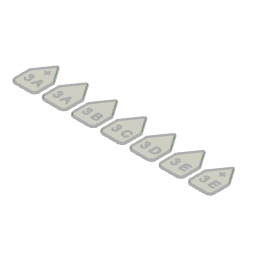
_Pointed Markers 3s.d0f4be62-6763-4f03-b29f-435d984270f3 (Autodesk Fusion 360 design; units mm, degrees)
Autodesk Fusion 360 part; units mm, degrees
sketch "Sketch1" plane through (0, 0, 0) normal (0, 0, 1) x (1, 0, 0)
  line L0 (0, 50.8) -> (0, 0)
  arc A0 (-31.7281, 6.3281) -> (-25.4, 0) centre (-25.4, 6.3281) ccw
  line L1 (-25.4, 0) -> (-15.875, 0)
  line L2 (-31.7281, 25.3781) -> (-31.7281, 6.3281)
  line L3 (-31.7281, 25.3781) -> (-15.7092, 48.2556)
  line L4 (-6.0183, 0) -> (-15.5433, 0)
  line L5 (0.3098, 25.3781) -> (-15.7092, 48.2556)
  arc A1 (-6.0183, 0) -> (0.3098, 6.3281) centre (-6.0183, 6.3281) ccw
  line L6 (0.3098, 25.3781) -> (0.3098, 6.3281)
  line L7 (-15.875, 0) -> (-15.5433, 0)
  dimension "d4" = 50.8
  dimension "d12" = 19.05
  constraint vertical L0
  constraint coincident L0.end origin
  constraint tangent A0 L1
  constraint vertical L2
  constraint parallel L4 L7
  measures "d4" distance of L0.end L0.start
  measures "d12" distance of A0.start L2.start
extrude "Extrude1" add sketch "Sketch1" along normal blind 1 contours L0 A0 L1 L2 L3 L4 L5 A1 L7 makes body 1
fillet "Fillet1" radius 2 3 edges at (0, 25.8206, 0.5) (-31.7281, 25.3781, 0.5) (-15.7092, 48.2556, 0.5) on bodies 1
sketch "Sketch2" plane through (0, 0, 1) normal (0, 0, 1) x (-1, 0, 0)
  arc A0 (14.0709, -45.9158) -> (17.3475, -45.9158) centre (15.7092, -44.7687) ccw
  line L0 (17.3475, -45.9158) -> (31.3664, -25.8947)
  arc A1 (31.3664, -25.8947) -> (31.7281, -24.7475) centre (29.7281, -24.7475) ccw
  line L1 (31.7281, -24.7475) -> (31.7281, -6.3281)
  arc A2 (31.7281, -6.3281) -> (25.4, 0) centre (25.4, -6.3281) ccw
  line L2 (25.4, 0) -> (6.0183, 0)
  arc A3 (6.0183, 0) -> (0, -4.3724) centre (6.0183, -6.3281) ccw
  line L3 (0, -4.3724) -> (0, -25.19)
  arc A4 (0, -25.19) -> (0.3617, -26.3371) centre (2, -25.19) ccw
  line L4 (0.3617, -26.3371) -> (14.0709, -45.9158)
  line L5 (16.1187, -45.0555) -> (30.1377, -25.0343)
  arc A5 (30.1377, -25.0343) -> (30.2281, -24.7475) centre (29.7281, -24.7475) ccw
  line L6 (30.2281, -24.7475) -> (30.2281, -6.3281)
  arc A6 (30.2281, -6.3281) -> (25.4, -1.5) centre (25.4, -6.3281) ccw
  line L7 (25.4, -1.5) -> (6.0183, -1.5)
  arc A7 (6.0183, -1.5) -> (1.5, -4.6265) centre (6.0183, -6.3281) ccw
  line L8 (1.5, -4.6265) -> (1.5, -25.19)
  arc A8 (1.5, -25.19) -> (1.5904, -25.4768) centre (2, -25.19) ccw
  line L9 (1.5904, -25.4768) -> (15.2996, -45.0555)
  arc A9 (15.2996, -45.0555) -> (16.1187, -45.0555) centre (15.7092, -44.7687) ccw
  line L10 (25.6864, -13.7884) -> (3.6261, -13.7884) construction
  line L11 (3.6261, -13.7884) -> (3.6261, -25.3842) construction
  line L12 (3.6261, -25.3842) -> (25.6864, -25.3842) construction
  line L13 (25.6864, -25.3842) -> (25.6864, -13.7884) construction
  dimension "d18" = -1.5
  dimension "d19" = 10.0076
copy_body "Body->Comp1" bodies 1 removing the originals makes body 2 in component "Arrow Base"
pattern_linear "R-Pattern1" count 1 spacing 0 along (0, 1, 0) count 7 spacing 38.1 along (1, 0, 0) of bodies 2 makes body 3 at (19.0573, 16.6458, 0) makes body 4 at (57.1573, 16.6458, 0) makes body 5 at (95.2573, 16.6458, 0) makes body 6 at (133.3573, 16.6458, 0) makes body 7 at (171.4573, 16.6458, 0) makes body 8 at (209.5573, 16.6458, 0) in component "Arrow Base"
sketch "Sketch3" plane through (0, 0, 1) normal (0, 0, 1) x (-1, 0, 0)
  arc A0 (14.0709, -45.9158) -> (17.3475, -45.9158) centre (15.7092, -44.7687) ccw
  line L0 (17.3475, -45.9158) -> (31.3664, -25.8947)
  arc A1 (31.3664, -25.8947) -> (31.7281, -24.7475) centre (29.7281, -24.7475) ccw
  line L1 (31.7281, -24.7475) -> (31.7281, -6.3281)
  arc A2 (31.7281, -6.3281) -> (25.4, 0) centre (25.4, -6.3281) ccw
  line L2 (25.4, 0) -> (6.0183, 0)
  arc A3 (6.0183, 0) -> (0, -4.3724) centre (6.0183, -6.3281) ccw
  line L3 (0, -4.3724) -> (0, -25.19)
  arc A4 (0, -25.19) -> (0.3617, -26.3371) centre (2, -25.19) ccw
  line L4 (0.3617, -26.3371) -> (14.0709, -45.9158)
  arc A5 (-24.0291, -45.9158) -> (-20.7525, -45.9158) centre (-22.3908, -44.7687) ccw
  line L5 (-20.7525, -45.9158) -> (-6.7336, -25.8947)
  arc A6 (-6.7336, -25.8947) -> (-6.3719, -24.7475) centre (-8.3719, -24.7475) ccw
  line L6 (-6.3719, -24.7475) -> (-6.3719, -6.3281)
  arc A7 (-6.3719, -6.3281) -> (-12.7, 0) centre (-12.7, -6.3281) ccw
  line L7 (-12.7, 0) -> (-32.0817, 0)
  arc A8 (-32.0817, 0) -> (-38.1, -4.3724) centre (-32.0817, -6.3281) ccw
  line L8 (-38.1, -4.3724) -> (-38.1, -25.19)
  arc A9 (-38.1, -25.19) -> (-37.7383, -26.3371) centre (-36.1, -25.19) ccw
  line L9 (-37.7383, -26.3371) -> (-24.0291, -45.9158)
  arc A10 (-62.1291, -45.9158) -> (-58.8525, -45.9158) centre (-60.4908, -44.7687) ccw
  line L10 (-58.8525, -45.9158) -> (-44.8336, -25.8947)
  arc A11 (-44.8336, -25.8947) -> (-44.4719, -24.7475) centre (-46.4719, -24.7475) ccw
  line L11 (-44.4719, -24.7475) -> (-44.4719, -6.3281)
  arc A12 (-44.4719, -6.3281) -> (-50.8, 0) centre (-50.8, -6.3281) ccw
  line L12 (-50.8, 0) -> (-70.1817, 0)
  arc A13 (-70.1817, 0) -> (-76.2, -4.3724) centre (-70.1817, -6.3281) ccw
  line L13 (-76.2, -4.3724) -> (-76.2, -25.19)
  arc A14 (-76.2, -25.19) -> (-75.8383, -26.3371) centre (-74.2, -25.19) ccw
  line L14 (-75.8383, -26.3371) -> (-62.1291, -45.9158)
  arc A15 (-100.2291, -45.9158) -> (-96.9525, -45.9158) centre (-98.5908, -44.7687) ccw
  line L15 (-96.9525, -45.9158) -> (-82.9336, -25.8947)
  arc A16 (-82.9336, -25.8947) -> (-82.5719, -24.7475) centre (-84.5719, -24.7475) ccw
  line L16 (-82.5719, -24.7475) -> (-82.5719, -6.3281)
  arc A17 (-82.5719, -6.3281) -> (-88.9, 0) centre (-88.9, -6.3281) ccw
  line L17 (-88.9, 0) -> (-108.2817, 0)
  arc A18 (-108.2817, 0) -> (-114.3, -4.3724) centre (-108.2817, -6.3281) ccw
  line L18 (-114.3, -4.3724) -> (-114.3, -25.19)
  arc A19 (-114.3, -25.19) -> (-113.9383, -26.3371) centre (-112.3, -25.19) ccw
  line L19 (-113.9383, -26.3371) -> (-100.2291, -45.9158)
  arc A20 (-138.3291, -45.9158) -> (-135.0525, -45.9158) centre (-136.6908, -44.7687) ccw
  line L20 (-135.0525, -45.9158) -> (-121.0336, -25.8947)
  arc A21 (-121.0336, -25.8947) -> (-120.6719, -24.7475) centre (-122.6719, -24.7475) ccw
  line L21 (-120.6719, -24.7475) -> (-120.6719, -6.3281)
  arc A22 (-120.6719, -6.3281) -> (-127, 0) centre (-127, -6.3281) ccw
  line L22 (-127, 0) -> (-146.3817, 0)
  arc A23 (-146.3817, 0) -> (-152.4, -4.3724) centre (-146.3817, -6.3281) ccw
  line L23 (-152.4, -4.3724) -> (-152.4, -25.19)
  arc A24 (-152.4, -25.19) -> (-152.0383, -26.3371) centre (-150.4, -25.19) ccw
  line L24 (-152.0383, -26.3371) -> (-138.3291, -45.9158)
  arc A25 (-176.4291, -45.9158) -> (-173.1525, -45.9158) centre (-174.7908, -44.7687) ccw
  line L25 (-173.1525, -45.9158) -> (-159.1336, -25.8947)
  arc A26 (-159.1336, -25.8947) -> (-158.7719, -24.7475) centre (-160.7719, -24.7475) ccw
  line L26 (-158.7719, -24.7475) -> (-158.7719, -6.3281)
  arc A27 (-158.7719, -6.3281) -> (-165.1, 0) centre (-165.1, -6.3281) ccw
  line L27 (-165.1, 0) -> (-184.4817, 0)
  arc A28 (-184.4817, 0) -> (-190.5, -4.3724) centre (-184.4817, -6.3281) ccw
  line L28 (-190.5, -4.3724) -> (-190.5, -25.19)
  arc A29 (-190.5, -25.19) -> (-190.1383, -26.3371) centre (-188.5, -25.19) ccw
  line L29 (-190.1383, -26.3371) -> (-176.4291, -45.9158)
  arc A30 (-214.5291, -45.9158) -> (-211.2525, -45.9158) centre (-212.8908, -44.7687) ccw
  line L30 (-211.2525, -45.9158) -> (-197.2336, -25.8947)
  arc A31 (-197.2336, -25.8947) -> (-196.8719, -24.7475) centre (-198.8719, -24.7475) ccw
  line L31 (-196.8719, -24.7475) -> (-196.8719, -6.3281)
  arc A32 (-196.8719, -6.3281) -> (-203.2, 0) centre (-203.2, -6.3281) ccw
  line L32 (-203.2, 0) -> (-222.5817, 0)
  arc A33 (-222.5817, 0) -> (-228.6, -4.3724) centre (-222.5817, -6.3281) ccw
  line L33 (-228.6, -4.3724) -> (-228.6, -25.19)
  arc A34 (-228.6, -25.19) -> (-228.2383, -26.3371) centre (-226.6, -25.19) ccw
  line L34 (-228.2383, -26.3371) -> (-214.5291, -45.9158)
  line L35 (16.1187, -45.0555) -> (30.1377, -25.0343)
  arc A35 (30.1377, -25.0343) -> (30.2281, -24.7475) centre (29.7281, -24.7475) ccw
  line L36 (30.2281, -24.7475) -> (30.2281, -6.3281)
  arc A36 (30.2281, -6.3281) -> (25.4, -1.5) centre (25.4, -6.3281) ccw
  line L37 (25.4, -1.5) -> (6.0183, -1.5)
  arc A37 (6.0183, -1.5) -> (1.5, -4.6265) centre (6.0183, -6.3281) ccw
  line L38 (1.5, -4.6265) -> (1.5, -25.19)
  arc A38 (1.5, -25.19) -> (1.5904, -25.4768) centre (2, -25.19) ccw
  line L39 (1.5904, -25.4768) -> (15.2996, -45.0555)
  arc A39 (15.2996, -45.0555) -> (16.1187, -45.0555) centre (15.7092, -44.7687) ccw
  line L40 (-21.9813, -45.0555) -> (-7.9623, -25.0343)
  arc A40 (-7.9623, -25.0343) -> (-7.8719, -24.7475) centre (-8.3719, -24.7475) ccw
  line L41 (-7.8719, -24.7475) -> (-7.8719, -6.3281)
  arc A41 (-7.8719, -6.3281) -> (-12.7, -1.5) centre (-12.7, -6.3281) ccw
  line L42 (-12.7, -1.5) -> (-32.0817, -1.5)
  arc A42 (-32.0817, -1.5) -> (-36.6, -4.6265) centre (-32.0817, -6.3281) ccw
  line L43 (-36.6, -4.6265) -> (-36.6, -25.19)
  arc A43 (-36.6, -25.19) -> (-36.5096, -25.4768) centre (-36.1, -25.19) ccw
  line L44 (-36.5096, -25.4768) -> (-22.8004, -45.0555)
  arc A44 (-22.8004, -45.0555) -> (-21.9813, -45.0555) centre (-22.3908, -44.7687) ccw
  line L45 (-60.0813, -45.0555) -> (-46.0623, -25.0343)
  arc A45 (-46.0623, -25.0343) -> (-45.9719, -24.7475) centre (-46.4719, -24.7475) ccw
  line L46 (-45.9719, -24.7475) -> (-45.9719, -6.3281)
  arc A46 (-45.9719, -6.3281) -> (-50.8, -1.5) centre (-50.8, -6.3281) ccw
  line L47 (-50.8, -1.5) -> (-70.1817, -1.5)
  arc A47 (-70.1817, -1.5) -> (-74.7, -4.6265) centre (-70.1817, -6.3281) ccw
  line L48 (-74.7, -4.6265) -> (-74.7, -25.19)
  arc A48 (-74.7, -25.19) -> (-74.6096, -25.4768) centre (-74.2, -25.19) ccw
  line L49 (-74.6096, -25.4768) -> (-60.9004, -45.0555)
  arc A49 (-60.9004, -45.0555) -> (-60.0813, -45.0555) centre (-60.4908, -44.7687) ccw
  line L50 (-98.1813, -45.0555) -> (-84.1623, -25.0343)
  arc A50 (-84.1623, -25.0343) -> (-84.0719, -24.7475) centre (-84.5719, -24.7475) ccw
  line L51 (-84.0719, -24.7475) -> (-84.0719, -6.3281)
  arc A51 (-84.0719, -6.3281) -> (-88.9, -1.5) centre (-88.9, -6.3281) ccw
  line L52 (-88.9, -1.5) -> (-108.2817, -1.5)
  arc A52 (-108.2817, -1.5) -> (-112.8, -4.6265) centre (-108.2817, -6.3281) ccw
  line L53 (-112.8, -4.6265) -> (-112.8, -25.19)
  arc A53 (-112.8, -25.19) -> (-112.7096, -25.4768) centre (-112.3, -25.19) ccw
  line L54 (-112.7096, -25.4768) -> (-99.0004, -45.0555)
  arc A54 (-99.0004, -45.0555) -> (-98.1813, -45.0555) centre (-98.5908, -44.7687) ccw
  line L55 (-136.2813, -45.0555) -> (-122.2623, -25.0343)
  arc A55 (-122.2623, -25.0343) -> (-122.1719, -24.7475) centre (-122.6719, -24.7475) ccw
  line L56 (-122.1719, -24.7475) -> (-122.1719, -6.3281)
  arc A56 (-122.1719, -6.3281) -> (-127, -1.5) centre (-127, -6.3281) ccw
  line L57 (-127, -1.5) -> (-146.3817, -1.5)
  arc A57 (-146.3817, -1.5) -> (-150.9, -4.6265) centre (-146.3817, -6.3281) ccw
  line L58 (-150.9, -4.6265) -> (-150.9, -25.19)
  arc A58 (-150.9, -25.19) -> (-150.8096, -25.4768) centre (-150.4, -25.19) ccw
  line L59 (-150.8096, -25.4768) -> (-137.1004, -45.0555)
  arc A59 (-137.1004, -45.0555) -> (-136.2813, -45.0555) centre (-136.6908, -44.7687) ccw
  line L60 (-160.2719, -24.7475) -> (-160.2719, -6.3281)
  arc A60 (-160.2719, -6.3281) -> (-165.1, -1.5) centre (-165.1, -6.3281) ccw
  line L61 (-165.1, -1.5) -> (-184.4817, -1.5)
  arc A61 (-184.4817, -1.5) -> (-189, -4.6265) centre (-184.4817, -6.3281) ccw
  line L62 (-189, -4.6265) -> (-189, -25.19)
  arc A62 (-189, -25.19) -> (-188.9096, -25.4768) centre (-188.5, -25.19) ccw
  line L63 (-188.9096, -25.4768) -> (-175.2004, -45.0555)
  arc A63 (-175.2004, -45.0555) -> (-174.3813, -45.0555) centre (-174.7908, -44.7687) ccw
  line L64 (-174.3813, -45.0555) -> (-160.3623, -25.0343)
  arc A64 (-160.3623, -25.0343) -> (-160.2719, -24.7475) centre (-160.7719, -24.7475) ccw
  line L65 (-212.4813, -45.0555) -> (-198.4623, -25.0343)
  arc A65 (-198.4623, -25.0343) -> (-198.3719, -24.7475) centre (-198.8719, -24.7475) ccw
  line L66 (-198.3719, -24.7475) -> (-198.3719, -6.3281)
  arc A66 (-198.3719, -6.3281) -> (-203.2, -1.5) centre (-203.2, -6.3281) ccw
  line L67 (-203.2, -1.5) -> (-222.5817, -1.5)
  arc A67 (-222.5817, -1.5) -> (-227.1, -4.6265) centre (-222.5817, -6.3281) ccw
  line L68 (-227.1, -4.6265) -> (-227.1, -25.19)
  arc A68 (-227.1, -25.19) -> (-227.0096, -25.4768) centre (-226.6, -25.19) ccw
  line L69 (-227.0096, -25.4768) -> (-213.3004, -45.0555)
  arc A69 (-213.3004, -45.0555) -> (-212.4813, -45.0555) centre (-212.8908, -44.7687) ccw
  line L70 (-7.9796, -5.9789) -> (-36.2077, -5.9789) construction
  line L71 (-36.2077, -5.9789) -> (-36.2077, -24.6143) construction
  line L72 (-36.2077, -24.6143) -> (-7.9796, -24.6143) construction
  line L73 (-7.9796, -24.6143) -> (-7.9796, -5.9789) construction
  line L74 (-46.2203, -6.1121) -> (-74.4484, -6.1121) construction
  line L75 (-74.4484, -6.1121) -> (-74.4484, -24.7475) construction
  line L76 (-74.4484, -24.7475) -> (-46.2203, -24.7475) construction
  line L77 (-46.2203, -24.7475) -> (-46.2203, -6.1121) construction
  line L78 (-84.8121, -6.1121) -> (-113.0403, -6.1121) construction
  line L79 (-113.0403, -6.1121) -> (-113.0403, -24.7475) construction
  line L80 (-113.0403, -24.7475) -> (-84.8121, -24.7475) construction
  line L81 (-84.8121, -24.7475) -> (-84.8121, -6.1121) construction
  line L82 (29.7281, -6.1121) -> (1.5, -6.1121) construction
  line L83 (1.5, -6.1121) -> (1.5, -24.7475) construction
  line L84 (1.5, -24.7475) -> (29.7281, -24.7475) construction
  line L85 (29.7281, -24.7475) -> (29.7281, -6.1121) construction
  line L86 (-122.5602, -5.9501) -> (-150.7883, -5.9501) construction
  line L87 (-150.7883, -5.9501) -> (-150.7883, -24.5855) construction
  line L88 (-150.7883, -24.5855) -> (-122.5602, -24.5855) construction
  line L89 (-122.5602, -24.5855) -> (-122.5602, -5.9501) construction
  line L90 (-160.6323, -6.4361) -> (-188.8604, -6.4361) construction
  line L91 (-188.8604, -6.4361) -> (-188.8604, -25.0715) construction
  line L92 (-188.8604, -25.0715) -> (-160.6323, -25.0715) construction
  line L93 (-160.6323, -25.0715) -> (-160.6323, -6.4361) construction
  line L94 (-199.0284, -6.1121) -> (-227.2565, -6.1121) construction
  line L95 (-227.2565, -6.1121) -> (-227.2565, -24.7475) construction
  line L96 (-227.2565, -24.7475) -> (-199.0284, -24.7475) construction
  line L97 (-199.0284, -24.7475) -> (-199.0284, -6.1121) construction
  line L98 (22.698, -27.7932) -> (8.8204, -27.7932) construction
  line L99 (8.8204, -27.7932) -> (8.8204, -35.5954) construction
  line L100 (8.8204, -35.5954) -> (22.698, -35.5954) construction
  line L101 (22.698, -35.5954) -> (22.698, -27.7932) construction
  line L102 (-205.8965, -27.4692) -> (-219.7741, -27.4692) construction
  line L103 (-219.7741, -27.4692) -> (-219.7741, -35.2714) construction
  line L104 (-219.7741, -35.2714) -> (-205.8965, -35.2714) construction
  line L105 (-205.8965, -35.2714) -> (-205.8965, -27.4692) construction
  dimension "d26" = -1.5
  dimension "d27" = -1.5
  dimension "d28" = -1.5
  dimension "d29" = -1.5
  dimension "d30" = -1.5
  dimension "d31" = -1.5
  dimension "d32" = -1.5
  dimension "d34" = 10.0076
  dimension "d35" = 10.0076
  dimension "d36" = 10.0076
  dimension "d37" = 10.0076
  dimension "d38" = 10.0076
  dimension "d39" = 10.0076
  dimension "d40" = 10.0076
  dimension "d41" = 10.0076
  dimension "d42" = 10.0076
  text T0 "3 A" font "Arial" height 10.0076 align centre middle in box 28.2281 x 18.6354 at (-7.9796, -5.9789) x (-1, 0) y (0, -1) spacing 1 kerned
  text T1 "3 B" font "Arial" height 10.0076 align centre middle in box 28.2281 x 18.6354 at (-46.2203, -6.1121) x (-1, 0) y (0, -1) spacing 1 kerned
  text T2 "3 C" font "Arial" height 10.0076 align centre middle in box 28.2281 x 18.6354 at (-84.8121, -6.1121) x (-1, 0) y (0, -1) spacing 1 kerned
  text T3 "3 A" font "Arial" height 10.0076 align centre middle in box 28.2281 x 18.6354 at (29.7281, -6.1121) x (-1, 0) y (0, -1) spacing 1 kerned
  text T4 "3 D" font "Arial" height 10.0076 align centre middle in box 28.2281 x 18.6354 at (-122.5602, -5.9501) x (-1, 0) y (0, -1) spacing 1 kerned
  text T5 "3 E" font "Arial" height 10.0076 align centre middle in box 28.2281 x 18.6354 at (-160.6323, -6.4361) x (-1, 0) y (0, -1) spacing 1 kerned
  text T6 "3 E" font "Arial" height 10.0076 align centre middle in box 28.2281 x 18.6354 at (-199.0284, -6.1121) x (-1, 0) y (0, -1) spacing 1 kerned
  text T7 "+\n" font "Arial" height 10.0076 align centre top in box 13.8776 x 7.8022 at (22.698, -27.7932) x (-1, 0) y (0, -1) spacing 1 kerned
  text T8 "+\n" font "Arial" height 10.0076 align centre top in box 13.8776 x 7.8022 at (-205.8965, -27.4692) x (-1, 0) y (0, -1) spacing 1 kerned
extrude "Extrude1'" add sketch "Sketch3" sketch "Sketch3" along normal blind 0.5 separate body of sketch 2 text T3 T4 T2 T7 T6 T8 T0 T5 T1 makes body 9 at (88.4257, 31.9948, 1) makes body 10 at (169.2987, 38.6685, 1) makes body 11 at (-21.6109, 38.9553, 1) makes body 12 at (213.0287, 29.5713, 1) makes body 13 at (-15.5658, 29.8953, 1) makes body 14 at (131.1987, 38.6685, 1) makes body 15 at (202.7257, 31.9948, 1) makes body 16 at (16.4891, 38.9553, 1) makes body 17 at (54.9987, 38.6685, 1) makes body 18 at (54.6093, 15.827, 1) makes body 19 at (16.372, 15.6937, 1) makes body 20 at (177.5429, 15.615, 1) makes body 21 at (-21.3357, 15.827, 1) makes body 22 at (-8.1846, 15.1317, 1) makes body 23 at (139.0544, 16.5421, 1) makes body 24 at (29.5231, 14.9985, 1) makes body 25 at (63.0456, 15.3024, 1) makes body 26 at (92.7199, 15.827, 1) makes body 27 at (130.5635, 15.665, 1) makes body 28 at (100.8868, 16.1043, 1) makes body 29 at (169.0247, 16.151, 1) makes body 30 at (215.939, 15.291, 1) makes body 31 at (207.4208, 15.827, 1) in component "Letters"
component "Letters" placed x (1, 0, 0) y (0, 1, 0) z (0, 0, 1) at (0, 0, 0)
component "Arrow Base" placed x (1, 0, 0) y (0, 1, 0) z (0, 0, 1) at (0, 0, 0)
equation "Num = 3"
equation "Num2 = 4"
